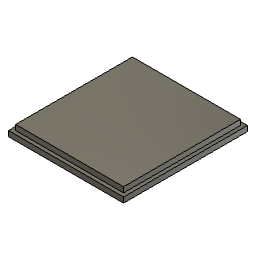
ensamble_pata (Autodesk Fusion 360 archive; units mm, degrees)
design "Tapa pata"
Autodesk Fusion 360 part; units mm, degrees
sketch "Sketch1" plane through (0, 0, 0) normal (0, 1, 0) x (1, 0, 0)
  line L0 (32.5, 35) -> (-32.5, 35)
  line L1 (-32.5, 35) -> (-32.5, -35)
  line L2 (-32.5, -35) -> (32.5, -35)
  line L3 (32.5, -35) -> (32.5, 35)
  line L4 (32.5, 35) -> (-32.5, -35) construction
  line L5 (-32.5, 35) -> (32.5, -35) construction
  dimension "d1" = 65
  dimension "d2" = 70
  constraint horizontal L0
  constraint perpendicular L0 L1
  constraint parallel L0 L2
  constraint parallel L1 L3
  constraint coincident L4 origin
  constraint coincident L5 origin
  measures "d1" distance of L1.end L2.end
  measures "d2" distance of L0.end L1.end
extrude "Extrude1" add sketch "Sketch1" along normal blind 3
sketch "Sketch2" plane through (0, 3, 0) normal (0, 1, 0) x (-1, 0, 0)
  line L0 (-32.5, 35) -> (-32.5, -35)
  line L1 (-32.5, -35) -> (32.5, -35)
  line L2 (32.5, -35) -> (32.5, 35)
  line L3 (32.5, 35) -> (-32.5, 35)
  line L4 (30.5, 33) -> (-30.5, 33)
  line L5 (-30.5, 33) -> (-30.5, -33)
  line L6 (-30.5, -33) -> (30.5, -33)
  line L7 (30.5, -33) -> (30.5, 33)
  line L8 (30.5, 33) -> (-30.5, -33) construction
  line L9 (-30.5, 33) -> (30.5, -33) construction
  dimension "d5" = 61
  dimension "d6" = 66
  constraint horizontal L4
  constraint perpendicular L4 L5
  constraint parallel L4 L6
  constraint parallel L5 L7
  constraint coincident L8 origin
  constraint coincident L9 origin
  measures "d5" distance of L5.end L6.end
  measures "d6" distance of L4.end L5.end
extrude "Extrude2" add sketch "Sketch2" along normal blind 3 contours L4 L5 L6 L7

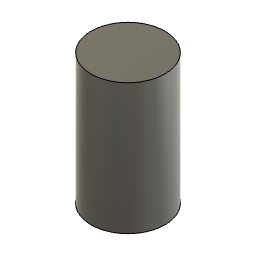
design "Pasador trasero"
Autodesk Fusion 360 part; units mm, degrees
sketch "Sketch1" plane through (0, 0, 0) normal (0, 1, 0) x (1, 0, 0)
  circle A0 centre (0, 0) radius 6
  dimension "d1" = 12
  constraint coincident A0.centre origin
  measures "d1" diameter of A0
extrude "Extrude1" add sketch "Sketch1" along normal blind 21.19

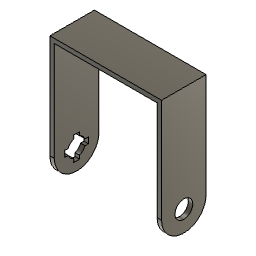
design "pierna"
Autodesk Fusion 360 part; units mm, degrees
sketch "Sketch1" plane through (0, 0, 0) normal (1, 0, 0) x (0, 1, 0)
  line L0 (0, 0) -> (30, 0)
  line L1 (30, 0) -> (30, 85)
  line L2 (30, 85) -> (0, 85)
  line L3 (0, 85) -> (0, 0)
  dimension "d1" = 30
  dimension "d32" = 85
  constraint horizontal L0
  constraint vertical L1
  constraint horizontal L2
  constraint vertical L3
  constraint coincident L0.start L3.end
  measures "d1" distance of L0.start L0.end
  measures "d32" distance of L0.start L2.end
extrude "Extrude1" add sketch "Sketch1" along normal blind 3
sketch "Sketch2" plane through (3, 0, 0) normal (1, 0, 0) x (0, 1, 0)
  line L0 (0, 85) -> (0, 0)
  line L1 (0, 0) -> (30, 0)
  line L2 (30, 0) -> (30, 85)
  line L3 (30, 85) -> (0, 85)
  point P0 (15, 11.8696)
  point P1 (15, 26.8696)
  dimension "d7" = 15
  measures "d7" distance of P0 P1
sketch "Sketch4" plane through (3, 0, 0) normal (1, 0, 0) x (0, 1, 0)
  line L0 (0, 85) -> (0, 0)
  line L1 (0, 0) -> (30, 0)
  line L2 (30, 0) -> (30, 85)
  line L3 (30, 85) -> (0, 85)
  circle A0 centre (15, 14) radius 6
  line L4 (17, 22) -> (13, 22)
  line L5 (13, 22) -> (13, 19.6569)
  line L6 (17, 19.6569) -> (17, 22)
  line L7 (17, 22) -> (13, 18) construction
  line L8 (13, 22) -> (17, 18) construction
  line L9 (7, 12) -> (9.3431, 12)
  line L10 (7, 16) -> (7, 12)
  line L11 (9.3431, 16) -> (7, 16)
  line L12 (17, 6) -> (17, 8.3431)
  line L13 (13, 6) -> (17, 6)
  line L14 (13, 8.3431) -> (13, 6)
  line L15 (23, 16) -> (20.6569, 16)
  line L16 (23, 12) -> (23, 16)
  line L17 (20.6569, 12) -> (23, 12)
  point P0 (15, 20)
  dimension "d16" = 12
  dimension "d17" = 14
  dimension "d18" = 15
  dimension "d19" = 4
  dimension "d20" = 4
  dimension "d22" = 360
  dimension "d23" = 2
  dimension "d24" = 8
  dimension "d25" = 2
  constraint horizontal L4
  constraint perpendicular L4 L5
  constraint parallel L5 L6
  constraint coincident L7 P0
  constraint coincident L8 P0
  constraint coincident A0 P0
  constraint coincident A0 L5.end
  constraint coincident A0 L6.start
  constraint perpendicular L7 L8
  measures "d16" diameter of A0
  measures "d17" vertical distance of L0.end A0.centre
  measures "d18" horizontal distance of L0.end A0.centre
  measures "d19" distance of L7.end L8.end
  measures "d20" distance of L4.end L7.end
  measures "d23" distance of L6 P0
  measures "d24" distance of A0.centre L4
  measures "d25" distance of L4 P0
extrude "Extrude3" cut sketch "Sketch4" against normal blind 3 contours A0 | A0 L15 L16 L17 | A0 L4 L5 L6 | A0 L12 L13 L14 | A0 L9 L10 L11
sketch "Sketch5" plane through (0, 0, 85) normal (0, 0, 1) x (-1, 0, 0)
  line L0 (0, -30) -> (0, 0)
  line L1 (0, 0) -> (-3, 0)
  line L2 (-3, 0) -> (-3, -30)
  line L3 (-3, -30) -> (0, -30)
  line L4 (0, -30) -> (-75.29, -30)
  line L5 (-75.29, -30) -> (-75.29, 0)
  line L6 (-75.29, 0) -> (0, 0)
  line L7 (0, 0) -> (0, -30)
  dimension "d28" = 75.29
  dimension "d29" = 30
  constraint horizontal L4
  constraint vertical L5
  constraint horizontal L6
  constraint vertical L7
  constraint coincident L0.start L3.end
  measures "d28" distance of L0.start L4.end
  measures "d29" distance of L0.start L0.end
extrude "Extrude4" add sketch "Sketch5" against normal blind 3 contours L2 L4 L5 L6
fillet "Fillet1" radius 15 2 edges at (1.5, 0, 0) (1.5, 30, 0)
sketch "Sketch6" plane through (0, 0, 82) normal (0, 0, -1) x (1, 0, 0)
  line L0 (75.29, -30) -> (75.29, 0)
  line L1 (75.29, 0) -> (3, 0)
  line L2 (3, 0) -> (3, -30)
  line L3 (3, -30) -> (75.29, -30)
  line L4 (75.29, 0) -> (72.29, 0)
  line L5 (72.29, 0) -> (72.29, -30)
  line L6 (72.29, -30) -> (75.29, -30)
  line L7 (75.29, -30) -> (75.29, 0)
  dimension "d37" = 3
  constraint horizontal L4
  constraint vertical L5
  constraint horizontal L6
  constraint vertical L7
  constraint coincident L0.end L1.start
  measures "d37" distance of L0.end L4.end
extrude "Extrude5" add sketch "Sketch6" along normal blind 82 contours L0 L1 L3 L4 L5 L6 L7
fillet "Fillet3" radius 15 2 edges at (73.79, 0, 0) (73.79, 30, 0)
sketch "Sketch7" plane through (75.29, 0, 0) normal (1, 0, 0) x (0, 1, 0)
  arc A0 (0, 15) -> (30, 15) centre (15, 15) ccw
  line L0 (30, 15) -> (30, 85)
  line L1 (30, 85) -> (0, 85)
  line L2 (0, 85) -> (0, 15)
  circle A1 centre (15, 14) radius 6
  dimension "d42" = 15
  dimension "d43" = 14
  dimension "d44" = 12
  measures "d42" horizontal distance of A1.centre origin
  measures "d43" vertical distance of A1.centre origin
  measures "d44" diameter of A1
extrude "Extrude6" cut sketch "Sketch7" against normal blind 10 contours A1

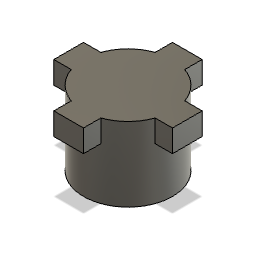
design "eje_pata"
Autodesk Fusion 360 part; units mm, degrees
sketch "Sketch1" plane through (0, 0, 0) normal (0, 1, 0) x (1, 0, 0)
  circle A0 centre (0, 0) radius 6
  dimension "d1" = 12
  constraint coincident A0.centre origin
  measures "d1" diameter of A0
extrude "Extrude1" add sketch "Sketch1" along normal blind 10
sketch "Sketch2" plane through (0, 10, 0) normal (0, 1, 0) x (-1, 0, 0)
  circle A0 centre (0, 0) radius 6
  line L0 (2, -8) -> (-2, -8)
  line L1 (-2, -8) -> (-2, -5.6569)
  line L2 (2, -5.6569) -> (2, -8)
  arc A1 (-2, -5.6569) -> (2, -5.6569) centre (0, 0) ccw
  dimension "d4" = 8
  dimension "d5" = 4
  dimension "d7" = 2
  constraint horizontal L0
  constraint vertical L1
  constraint vertical L2
  constraint coincident A0 L2.start
  constraint coincident A0 L1.end
  constraint coincident A0.centre A1.centre
  measures "d4" distance of A0.centre L0
  measures "d5" distance of L1 L2
  measures "d7" distance of A0.centre L1
extrude "Extrude2" add sketch "Sketch2" against normal blind 3 contours A0 L0 L1 L2 A1
pattern_circular "C-Pattern1" count 4 over 360 about axis through (0, 1.75, 0) along (0, 1, 0) of "Extrude2"

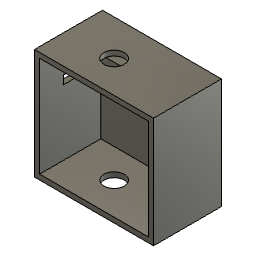
design "base_pata"
Autodesk Fusion 360 part; units mm, degrees
sketch "Sketch1" plane through (0, 0, 0) normal (0, 0, 1) x (1, 0, 0)
  line L0 (0, 0) -> (70, 0)
  line L1 (70, 0) -> (70, 65)
  line L2 (70, 65) -> (0, 65)
  line L3 (0, 65) -> (0, 0)
  dimension "d1_1" = 70
  dimension "d2_1" = 65
  constraint horizontal L0
  constraint vertical L1
  constraint horizontal L2
  constraint vertical L3
  constraint coincident L0.start L3.end
  measures "d1_1" distance of L0.start L0.end
  measures "d2_1" distance of L0.start L2.end
extrude "Extrude1" add sketch "Sketch1" along normal blind 40
shell "Shell1" thickness 3 removed faces 1 at (23.3333, 43.3333, 40)
sketch "Sketch3" plane through (0, 0, 3) normal (0, 0, 1) x (-1, 0, 0)
  line L0 (-3, -3) -> (-67, -3)
  line L1 (-67, -3) -> (-67, -62)
  line L2 (-67, -62) -> (-3, -62)
  line L3 (-3, -62) -> (-3, -3)
  line L4 (-10, -52.9161) -> (-60, -52.9161)
  line L5 (-60, -52.9161) -> (-60, -10)
  line L6 (-60, -10) -> (-10, -10)
  line L7 (-10, -10) -> (-10, -52.9161)
  dimension "d13" = 7
  dimension "d14" = 7
  dimension "d15" = 50
  constraint horizontal L4
  constraint vertical L5
  constraint horizontal L6
  constraint vertical L7
  measures "d13" distance of L0 L6
  measures "d14" distance of L3 L7
  measures "d15" distance of L5.end L6.end
extrude "Extrude2" add sketch "Sketch3" along normal blind 8 contours L4 L5 L6 L7
sketch "Sketch4" plane through (0, 0, 0) normal (0, -1, 0) x (1, 0, 0)
  line L0 (0, 0) -> (70, 0)
  line L1 (70, 0) -> (70, 40)
  line L2 (70, 40) -> (0, 40)
  line L3 (0, 40) -> (0, 0)
  circle A0 centre (28, 21.15) radius 6
  dimension "d8" = 21.15
  dimension "d9" = 28
  dimension "d10" = 12
  measures "d8" vertical distance of L0.start A0.centre
  measures "d9" horizontal distance of L0.start A0.centre
  measures "d10" diameter of A0
extrude "Extrude3" cut sketch "Sketch4" against normal blind 65 contours A0
sketch "Sketch5" plane through (0, 0, 0) normal (-1, 0, 0) x (0, 0, 1)
  line L0 (0, 65) -> (0, 0)
  line L1 (0, 0) -> (40, 0)
  line L2 (40, 0) -> (40, 65)
  line L3 (40, 65) -> (0, 65)
  line L4 (16, 46.5) -> (26, 46.5)
  line L5 (26, 46.5) -> (26, 41.5)
  line L6 (26, 41.5) -> (16, 41.5)
  line L7 (16, 41.5) -> (16, 46.5)
  dimension "d16" = 16
  dimension "d17" = 18.5
  dimension "d18" = 10
  dimension "d19" = 5
  constraint horizontal L4
  constraint vertical L5
  constraint horizontal L6
  constraint vertical L7
  measures "d16" horizontal distance of L0.start L4.start
  measures "d17" vertical distance of L0.start L4.start
  measures "d18" distance of L4.start L4.end
  measures "d19" distance of L4.start L6.end
extrude "Extrude4" cut sketch "Sketch5" against normal blind 3 contours L4 L5 L6 L7
